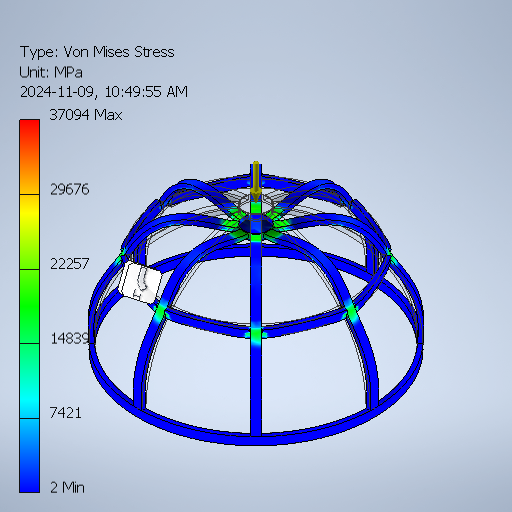
# Autodesk Inventor part: Dome
Saved by Autodesk Inventor 2025.1 (Build 291241000, 241)
## iProperties
Created: 2024-11-07
Part Number: Dome
Material: Steel, Mild
Document SubType Name: Modeling
Designer: smonowar1008
Density: 7.85 g/cm^3
Appearance: Semi-Polished
Author: smonowar1008
Autodesk Inventor part; units mm, degrees
sketch "Sketch1" plane through (0, 0, 0) normal (0, 1, 0) x (-1, 0, 0)
  circle A0 centre (0, 0) radius 95
  circle A1 centre (0, 0) radius 91.825
  dimension "d0" = 190
  dimension "d1" = 183.65
  constraints: 2 centre point, 2 coincident
  measures "d0" diameter of A0
  measures "d1" diameter of A1
extrude "Extrusion1" add sketch "Sketch1" along normal blind 6.35
sketch "Sketch2" plane through (0, 0, 0) normal (1, 0, 0) x (0, 1, 0)
  line L0 (6.35, -95) -> (6.35, 95) projected
  arc A0 (101.35, 0) -> (6.35, 95) centre (6.35, 0) ccw
  arc A1 (98.175, 0) -> (6.35, 91.825) centre (6.35, 0) ccw
  line L1 (101.35, 0) -> (98.175, 0)
  line L2 (6.35, 95) -> (6.35, 91.825)
  point P0 (0, 0)
  dimension "d11" = 91.825
  constraints: 4 end point, 4 point on circle, 2 centre point, 1 coincident, 1 collinear, 1 horizontal, 1 midpoint, 1 point on line
  measures "d11" radius of A1
extrude "Curved Bar 1" add sketch "Sketch2" along normal mid plane 6.35
sketch "Sketch4" plane through (0, 0, 0) normal (1, 0, 0) x (0, 1, 0)
  line L0 (6.35, -95) -> (6.35, 95) projected
  arc A0 (6.35, -95) -> (101.35, 0) centre (6.35, 0) ccw
  arc A1 (6.35, -91.825) -> (98.175, 0) centre (6.35, 0) ccw
  line L1 (101.35, 0) -> (98.175, 0)
  line L2 (6.35, -95) -> (6.35, -91.825)
  point P0 (0, 0)
  point P1 (6.35, 94.9469)
  dimension "d18" = 91.825
  constraints: 4 end point, 4 point on circle, 2 centre point, 1 coincident, 1 horizontal, 1 midpoint, 1 perpendicular
  measures "d18" radius of A1
extrude "Extrusion4" add sketch "Sketch4" along normal mid plane 6.35
sketch "Sketch5" plane through (0, 0, 0) normal (0, 0, 1) x (1, 0, 0)
  line L0 (0, 6.35) -> (-3.175, 6.35) projected
  line L1 (-3.175, 101.35) -> (3.175, 101.35) projected
  line L2 (-3.175, 6.35) -> (-95, 6.35) projected
  arc A0 (0, 101.35) -> (-95, 6.35) centre (0, 6.35) ccw
  arc A1 (0, 98.175) -> (-91.825, 6.35) centre (0, 6.35) ccw
  line L3 (0, 101.35) -> (0, 98.175)
  line L4 (-91.825, 6.35) -> (-95, 6.35)
  point P0 (0, 0)
  point P1 (-91.825, 6.35)
  dimension "d21" = 91.825
  constraints: 4 end point, 4 point on circle, 2 centre point, 1 coincident, 1 midpoint, 1 perpendicular, 1 vertical
  measures "d21" radius of A1
extrude "Extrusion5" add sketch "Sketch5" along normal mid plane 6.35
sketch "Sketch6" plane through (0, 0, 0) normal (0, 0, 1) x (1, 0, 0)
  line L0 (0, 6.35) -> (-3.175, 6.35) projected
  line L1 (95, 6.35) -> (3.175, 6.35) projected
  line L2 (0, 101.2969) -> (0, 101.35) projected
  arc A0 (95, 6.35) -> (0, 101.35) centre (0, 6.35) ccw
  line L3 (0, 6.35) -> (91.825, 6.35) projected
  arc A1 (91.825, 6.35) -> (0, 98.175) centre (0, 6.35) ccw
  line L4 (95, 6.35) -> (91.825, 6.35)
  line L5 (0, 101.35) -> (0, 98.175)
  point P0 (0, 0)
  dimension "d24" = 91.825
  constraints: 5 point on circle, 4 end point, 2 centre point, 1 coincident, 1 horizontal, 1 perpendicular, 1 point on line
  measures "d24" radius of A1
extrude "Extrusion6" add sketch "Sketch6" along normal mid plane 6.35
ref_plane "Work Plane2" through (0, 0, 0) normal (0.7071068, 0, -0.7071068) x (0, 1, 0)
sketch "Sketch9" plane through (0, 0, 0) normal (0.7071068, 0, -0.7071068) x (0, 1, 0)
  line L0 (6.35, 64.9301) -> (6.35, -64.9301) projected
  line L1 (0, 95) -> (6.35, 95) projected
  arc A0 (101.35, 0) -> (6.35, 95) centre (6.35, 0) ccw
  arc A1 (98.175, 0) -> (6.35, 91.825) centre (6.35, 0) ccw
  line L2 (101.35, 0) -> (98.175, 0)
  line L3 (6.35, 95) -> (6.35, 91.825)
  point P0 (0, 0)
  dimension "d35" = 91.825
  constraints: 4 end point, 4 point on circle, 2 centre point, 1 coincident, 1 horizontal, 1 midpoint, 1 perpendicular, 1 point on line
  measures "d35" radius of A1
extrude "Extrusion9" add sketch "Sketch9" along normal mid plane 6.35
sketch "Sketch10" plane through (0, 0, 0) normal (0.7071068, 0, -0.7071068) x (0, 1, 0)
  line L0 (6.35, -64.8926) -> (6.35, 64.8926) projected
  line L1 (6.35, -95) -> (6.35, -69.3827) projected
  arc A0 (6.35, -95) -> (101.35, 0) centre (6.35, 0) ccw
  line L2 (6.35, 0) -> (101.35, 0) construction
  line L3 (6.35, 0) -> (6.35, -95) construction
  arc A1 (6.35, -91.825) -> (98.175, 0) centre (6.35, 0) ccw
  line L4 (101.2969, 0) -> (101.3235, 0) projected
  line L5 (101.35, 0) -> (98.175, 0)
  line L6 (6.35, -95) -> (6.35, -91.825)
  point P0 (0, 0)
  dimension "d38" = 95
  dimension "d39" = 90
  dimension "d40" = 91.825
  constraints: 8 end point, 4 point on circle, 2 centre point, 2 point on line, 1 coincident, 1 midpoint
  measures "d38" radius of A0
  measures "d39" angle of L3 L2
  measures "d40" radius of A1
extrude "Extrusion10" add sketch "Sketch10" along normal mid plane 6.35
ref_plane "Work Plane8" through (-67.1751, 6.35, 67.1751) normal (-0.7071068, 0, -0.7071068) x (0, -1, 0)
sketch "Sketch14" plane through (-67.1751, 6.35, 67.1751) normal (-0.7071068, 0, -0.7071068) x (0, -1, 0)
  line L0 (0, -95) -> (0, -30.0699)
  line L1 (0, 0) -> (0, -25.6173)
  arc A0 (0, 0) -> (-95, -95) centre (0, -95) ccw
  ellipse E0 centre (0, -95) end of major axis (-91.825, -95) minor radius 38.0352 (-91.5045, -91.825) -> (-91.825, -95) ccw
  arc A1 (0, -3.175) -> (-91.825, -95) centre (0, -95) ccw
  line L2 (-95, -95) -> (-91.825, -95)
  line L3 (0, -3.175) -> (0, 0)
  ellipse E1 centre (0, -97.2451) end of major axis (91.825, -97.2451) minor radius 64.9301 (-91.7701, -99.4901) -> (0, -162.1751) ccw
  arc A2 (-95, -95) -> (0, -190) centre (0, -95) ccw
  line L4 (0, -186.825) -> (0, -159.9301)
  arc A3 (-91.825, -95) -> (0, -186.825) centre (0, -95) ccw
  line L5 (-91.825, -95) -> (-95, -95)
  line L6 (0, -190) -> (0, -186.825)
  point P0 (6.35, -95)
  dimension "d51" = 91.825
  dimension "d52" = 91.825
  constraints: 14 end point, 8 point on circle, 4 centre point, 3 coincident, 3 point on line, 8 other
  measures "d51" radius of A1
  measures "d52" radius of A3
extrude "Extrusion13" add sketch "Sketch14" along normal mid plane 6.35 contours L1 A1 L2 A0
extrude "Extrusion14" add sketch "Sketch14" along normal mid plane 6.35 contours L2 A3 L6 A2
ref_plane "Work Plane9" through (0, 101.35, 0) normal (0, 1, 0) x (-1, 0, 0)
sketch "Sketch15" plane through (0, 101.35, 0) normal (0, 1, 0) x (-1, 0, 0)
  circle A0 centre (0, 0) radius 10
  dimension "d57" = 20
  constraints: 1 centre point, 1 coincident
  measures "d57" diameter of A0
extrude "Extrusion15" add sketch "Sketch15" against normal blind 5.08
ref_plane "Work Plane11" through (0, 65, 0) normal (0, 1, 0) x (-1, 0, 0)
sketch "Sketch17" plane through (0, 65, 0) normal (0, 1, 0) x (-1, 0, 0)
  line L0 (3.175, 9.4826) -> (3.175, 95) projected
  line L1 (3.175, 74.4323) -> (3.175, 71.2543)
  line L2 (-3.175, 71.2543) -> (-3.175, 74.4323)
  line L3 (-4.4601, 8.9503) -> (-64.9301, 69.4202) projected
  arc A0 (-3.175, 71.2543) -> (-48.1393, 52.6295) centre (0, 0) ccw
  arc A1 (-3.175, 74.4323) -> (-50.3865, 54.8767) centre (0, 0) ccw
  line L4 (-91.825, 3.175) -> (-9.4826, 3.175) projected
  line L5 (-71.2543, 3.175) -> (-74.4323, 3.175)
  line L6 (-95, -3.175) -> (-9.4826, -3.175) projected
  line L7 (-71.2543, -3.175) -> (-74.4323, -3.175)
  arc A2 (-54.8767, 50.3865) -> (-74.4323, 3.175) centre (0, 0) ccw
  arc A3 (-52.6295, 48.1393) -> (-71.2543, 3.175) centre (0, 0) ccw
  line L8 (-67.1751, -62.685) -> (-8.9503, -4.4601) projected
  line L9 (-54.8767, -50.3865) -> (-52.6295, -48.1393)
  line L10 (-50.3865, -54.8767) -> (-48.1393, -52.6295)
  arc A4 (-71.2543, -3.175) -> (-52.6295, -48.1393) centre (0, 0) ccw
  arc A5 (-74.4323, -3.175) -> (-54.8767, -50.3865) centre (0, 0) ccw
  line L11 (-3.175, -91.825) -> (-3.175, -9.4826) projected
  line L12 (-3.175, -71.2543) -> (-3.175, -74.4323)
  line L13 (3.175, -74.4323) -> (3.175, -71.2543)
  arc A6 (-48.1393, -52.6295) -> (-3.175, -71.2543) centre (0, 0) ccw
  arc A7 (-50.3865, -54.8767) -> (-3.175, -74.4323) centre (0, 0) ccw
  arc A8 (3.175, -71.2543) -> (48.1393, -52.6295) centre (0, 0) ccw
  arc A9 (3.175, -74.4323) -> (50.3865, -54.8767) centre (0, 0) ccw
  line L14 (48.1393, -52.6295) -> (50.3865, -54.8767)
  line L15 (4.4601, -8.9503) -> (64.9301, -69.4202) projected
  line L16 (52.6295, -48.1393) -> (54.8767, -50.3865)
  line L17 (69.4202, -64.9301) -> (8.9503, -4.4601) projected
  arc A10 (52.6295, -48.1393) -> (71.2543, -3.175) centre (0, 0) ccw
  arc A11 (54.8767, -50.3865) -> (74.4323, -3.175) centre (0, 0) ccw
  line L18 (71.2543, -3.175) -> (74.4323, -3.175)
  line L19 (9.4826, -3.175) -> (95, -3.175) projected
  line L20 (71.2543, 3.175) -> (74.4323, 3.175)
  line L21 (95, 3.175) -> (9.4826, 3.175) projected
  arc A12 (71.2543, 3.175) -> (52.6295, 48.1393) centre (0, 0) ccw
  arc A13 (48.1393, 52.6295) -> (3.175, 71.2543) centre (0, 0) ccw
  arc A14 (74.4323, 3.175) -> (54.8767, 50.3865) centre (0, 0) ccw
  arc A15 (50.3865, 54.8767) -> (3.175, 74.4323) centre (0, 0) ccw
  line L22 (52.6295, 48.1393) -> (54.8767, 50.3865)
  line L23 (8.9503, 4.4601) -> (69.4202, 64.9301) projected
  line L24 (48.1393, 52.6295) -> (50.3865, 54.8767)
  line L25 (-50.3865, 54.8767) -> (-48.1393, 52.6295)
  line L26 (-52.6295, 48.1393) -> (-54.8767, 50.3865)
  line L27 (-8.9503, 4.4601) -> (-67.1751, 62.685) projected
  point P0 (-48.1178, 52.6492)
  constraints: 33 point on circle, 32 end point, 22 point on line, 16 centre point, 7 collinear, 4 parallel, 2 coincident
extrude "Extrusion17" add sketch "Sketch17" along normal mid plane 6.35 contours A0 L3 A1 L2
extrude "Extrusion18" add sketch "Sketch17" along normal mid plane 6.35 contours L0 A15 L24 A13 | A2 L26 A3 L4 | L6 A4 L8 A5 | L10 A6 L11 A7 | L13 A8 L14 A9 | A10 L18 A11 L16 | A12 L22 A14 L20
body "Solid1"
